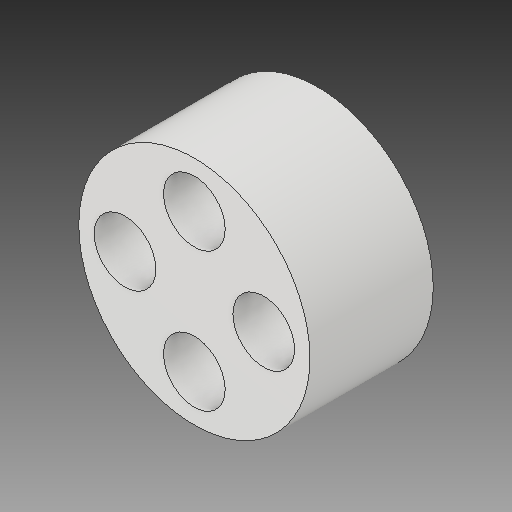
# Autodesk Inventor part: アーム中間節カム2
Saved by Autodesk Inventor 2020 (Build 240168000, 168)
## iProperties
Created: 2018-11-21
Part Number: アーム中間節カム2
Material: アセタール樹脂、白
Document SubType Name: Modeling
Designer: 雪村
Density: 1.425 g/cm^3
Appearance: 滑らか - 白
Mass: 1.44152 g
Surface Area: 10.3201 cm^2
Volume: 1.01159 cm^3
Description: ジュラコン 8t
Author: 雪村
Autodesk Inventor part; units mm, degrees
ref_plane "YZ Plane" through (0, 0, 0) normal (1, 0, 0) x (0, 1, 0)
ref_plane "XZ Plane" through (0, 0, 0) normal (0, 1, 0) x (-1, 0, 0)
ref_plane "XY Plane" through (0, 0, 0) normal (0, 0, 1) x (1, 0, 0)
sketch "スケッチ1" plane through (0, 0, 0) normal (0, 0, 1) x (1, 0, 0)
  circle A0 centre (0, 0) radius 7.5
  circle A1 centre (-4.5, 0) radius 4.5 construction
  circle A2 centre (4.5, 0) radius 4.5 construction
  circle A3 centre (-4.5, 0) radius 2
  circle A4 centre (4.5, 0) radius 2
  dimension "d1" = 9
  dimension "d0" = 15
  dimension "d2" = 9
  dimension "d3" = 4
  dimension "d4" = 4
  constraints: 4 centre point, 3 coincident, 3 horizontal alignment, 3 other
  measures "d0" diameter of A0
  measures "d2" diameter of A2
  measures "d3" diameter of A3
  measures "d4" diameter of A4
extrude "押し出し1" add sketch "スケッチ1" along normal blind 8
sketch "スケッチ2" plane through (0, 0, 8) normal (0, 0, 1) x (1, 0, 0)
  line L0 (0, 4.5) -> (4.5, 0)
  line L1 (4.5, 0) -> (0, -4.5)
  line L2 (0, -4.5) -> (-4.5, 0)
  line L3 (-4.5, 0) -> (0, 4.5)
  circle A0 centre (4.5, 0) radius 2 projected
  circle A1 centre (0, 4.5) radius 2
  circle A2 centre (0, -4.5) radius 2
  point P0 (0, 0)
  point P1 (0, 0)
  dimension "d7" = 4
  dimension "d8" = 4
  constraints: 8 end point, 4 coincident, 2 centre point, 9 other
  measures "d7" diameter of A1
  measures "d8" diameter of A2
extrude "押し出し2" cut sketch "スケッチ2" against normal through all contours L3 A1 L0 | L0 A1 L3 | A2 L1 L2 | L2 L1 A2
